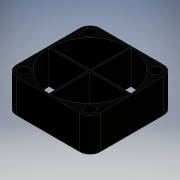
# Autodesk Inventor part: Fan
Saved by Autodesk Inventor 2016 (Build 200138000, 138)
## iProperties
Created: 2019-09-20
Part Number: Fan
Material: Generic
Document SubType Name: Modeling
Designer: jimmy
Density: 1 g/cm^3
Appearance: Default
Author: jimmy
Autodesk Inventor part; units mm, degrees
ref_plane "YZ Plane" through (0, 0, 0) normal (1, 0, 0) x (0, 1, 0)
ref_plane "XZ Plane" through (0, 0, 0) normal (0, 1, 0) x (-1, 0, 0)
ref_plane "XY Plane" through (0, 0, 0) normal (0, 0, 1) x (1, 0, 0)
sketch "Sketch1" plane through (0, 0, 0) normal (0, 0, 1) x (1, 0, 0)
  line L0 (-12.5, -12.5) -> (12.5, -12.5)
  line L1 (12.5, -12.5) -> (12.5, 12.5)
  line L2 (12.5, 12.5) -> (-12.5, 12.5)
  line L3 (-12.5, 12.5) -> (-12.5, -12.5)
  line L4 (-12.5, -12.5) -> (12.5, 12.5) construction
  line L5 (12.5, -12.5) -> (-12.5, 12.5) construction
  point P0 (0, 0)
  dimension "d0" = 25
  dimension "d1" = 25
  constraints: 12 end point, 2 midpoint, 2 parallel, 1 horizontal, 1 perpendicular
  measures "d0" distance of L2.end L1.end
  measures "d1" distance of L1.end L0.end
extrude "Extrusion1" add sketch "Sketch1" along normal blind 10
sketch "Sketch2" plane through (0, 0, 10) normal (0, 0, 1) x (1, 0, 0)
  circle A0 centre (0, 0) radius 14 construction
  line L0 (0, 0) -> (-9.8995, 9.8995) construction
  line L1 (-19.6, 0) -> (19.6, 0) construction
  line L2 (0, -19.6) -> (0, 19.6) construction
  point P0 (-9.8995, -9.8995)
  point P1 (9.8995, -9.8995)
  point P2 (9.8995, 9.8995)
  dimension "d4" = 28
  dimension "d5" = 45
  dimension "d8" = 360
  constraints: 2 coincident, 2 end point, 8 other
  measures "d5" angle of L0 L2
hole "Hole1" at (-9.8995, 9.8995, 10) at (-9.8995, -9.8995, 10) at (9.8995, -9.8995, 10) at (9.8995, 9.8995, 10) direction (0, 0, -1) diameter 3 depth 15.25 tip angle 118
fillet "Fillet1" radius 3 4 edges at (-12.5, 12.5, 5) (12.5, 12.5, 5) (12.5, -12.5, 5) (-12.5, -12.5, 5)
sketch "Sketch3" plane through (0, 0, 10) normal (0, 0, 1) x (1, 0, 0)
  circle A0 centre (0, 0) radius 12
  dimension "d18" = 24
  constraints: 1 centre point, 1 coincident
  measures "d18" diameter of A0
extrude "Extrusion2" cut sketch "Sketch3" against normal blind 10
sketch "Sketch4" plane through (0, 0, 10) normal (0, 0, 1) x (1, 0, 0)
  line L0 (-12.2062, -0.25) -> (12.2062, -0.25)
  line L1 (12.2062, -0.25) -> (12.2062, 0.25)
  line L2 (12.2062, 0.25) -> (-12.2062, 0.25)
  line L3 (-12.2062, 0.25) -> (-12.2062, -0.25)
  line L4 (-12.2062, -0.25) -> (12.2062, 0.25) construction
  line L5 (12.2062, -0.25) -> (-12.2062, 0.25) construction
  line L6 (-0.25, -12.2062) -> (0.25, -12.2062)
  line L7 (0.25, -12.2062) -> (0.25, 12.2062)
  line L8 (0.25, 12.2062) -> (-0.25, 12.2062)
  line L9 (-0.25, 12.2062) -> (-0.25, -12.2062)
  circle A0 centre (0, 0) radius 12 projected
  line L10 (-0.25, -12.2062) -> (0.25, 12.2062) construction
  line L11 (0.25, -12.2062) -> (-0.25, 12.2062) construction
  dimension "d21" = 0.5
  dimension "d22" = 0.5
  constraints: 24 end point, 4 midpoint, 4 parallel, 2 horizontal, 2 perpendicular
  measures "d21" distance of L1.end L0.end
  measures "d22" distance of L8.end L7.end
extrude "Extrusion3" add sketch "Sketch4" against normal blind 10 contours L3 L2 A0 L0 | A0 L2 L9 L0 | L9 L2 L7 L0 | L0 L7 A0 L9 | A0 L7 L6 L9 | L7 L2 A0 L0 | L9 A0 L7 L2 | L9 L8 L7 A0 | A0 L2 L1 L0
body "Solid1"
